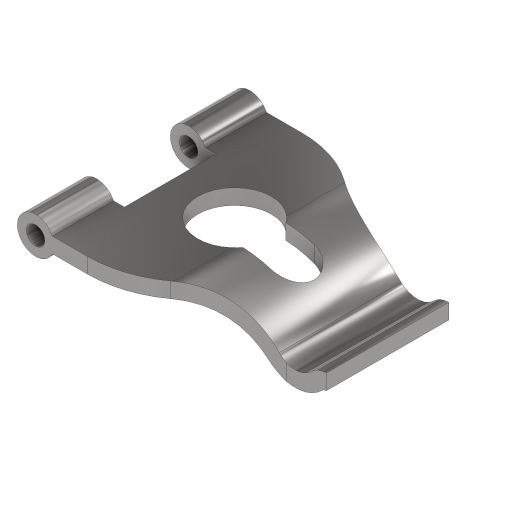
# Autodesk Inventor part: Part017. Tilting clamo
Saved by Autodesk Inventor 2023.2 (Build 272271030, 271C)
## iProperties
Created: 2023-09-19
Part Number: Part017. Tilting clamo
Material: Steel, Carbon
Document SubType Name: Modeling
Designer: User
Mass: 160.607 g
Surface Area: 109.731 cm^2
Volume: 20.4595 cm^3
Density: 7.85 g/cm^3
Appearance: Steel - Polished
Author: User
Autodesk Inventor part; units mm, degrees
ref_plane "YZ Plane" through (0, 0, 0) normal (1, 0, 0) x (0, 1, 0)
ref_plane "XZ Plane" through (0, 0, 0) normal (0, 1, 0) x (-1, 0, 0)
ref_plane "XY Plane" through (0, 0, 0) normal (0, 0, 1) x (1, 0, 0)
sketch "Sketch1" plane through (0, 0, 0) normal (0, 0, 1) x (1, 0, 0)
  line L0 (0, 0) -> (38, 0) construction
  arc A0 (62.7487, -10.2513) -> (38, 0) centre (38, -35) ccw construction
  arc A1 (62.7487, -10.2513) -> (76.8909, -10.2513) centre (69.8198, -3.1802) ccw construction
  arc A2 (80, -8.9625) -> (76.8909, -10.2513) centre (80.0021, -13.3625) ccw construction
  line L1 (38, 0) -> (38, -35) construction
  line L2 (38, -35) -> (69.8198, -3.1802) construction
  line L3 (69.8198, -3.1802) -> (80.0021, -13.3625) construction
  line L4 (5.4544, 2.5) -> (38, 2.5)
  arc A3 (64.5165, -8.4835) -> (38, 2.5) centre (38, -35) ccw
  arc A4 (64.5165, -8.4835) -> (75.1231, -8.4835) centre (69.8198, -3.1802) ccw
  arc A5 (79.9988, -6.4625) -> (75.1231, -8.4835) centre (80.0021, -13.3625) ccw
  arc A6 (60.981, -12.019) -> (38, -2.5) centre (38, -35) ccw
  arc A7 (60.981, -12.019) -> (78.6586, -12.019) centre (69.8198, -3.1802) ccw
  arc A8 (79.9988, -11.4625) -> (78.6586, -12.019) centre (80.0021, -13.3625) ccw
  line L5 (79.9988, -6.4625) -> (79.9988, -11.4625)
  arc A9 (5.4544, 2.5) -> (5.4544, -2.5) centre (0, 0) ccw
  circle A10 centre (0, 0) radius 3
  line L6 (5.4544, -2.5) -> (38, -2.5)
  dimension "d0" = 38
  dimension "d1" = 35
  dimension "d2" = 10
  dimension "d3" = 4.4
  dimension "d4" = 45
  dimension "d5" = 80
  dimension "d6" = 2.5
  dimension "d8" = 12
  dimension "d9" = 6
  constraints: 20 point on circle, 14 end point, 11 centre point, 3 tangent, 2 coincident, 2 vertical, 1 horizontal, 1 perpendicular, 4 other
  measures "d0" distance of L0.start L0.end
  measures "d1" radius of A0
  measures "d2" radius of A1
  measures "d3" radius of A2
  measures "d4" angle of L2 L1
  measures "d5" horizontal distance of A2.start L0.start
  measures "d6" distance between parallel lines of L0 L4
  measures "d8" diameter of A9
  measures "d9" diameter of A10
extrude "Extrusion1" add sketch "Sketch1" along normal mid plane 70
fillet "Fillet1" radius 3 2 edges at (79.9988, -8.9625, 35) (79.9988, -8.9625, -35)
sketch "Sketch2" plane through (0, 0, 0) normal (0, 1, 0) x (-1, 0, 0)
  line L0 (6, -35) -> (6, 35) projected
  line L1 (-79.9988, -32) -> (-79.9988, 32) projected
  line L2 (23.2007, 0) -> (-97.2041, 0) construction
  line L3 (6, 35) -> (-5.4544, 35) construction
  line L4 (6, 35) -> (-17, 35)
  arc A0 (-17, 35) -> (-37.4698, 28.3899) centre (-17, 0) ccw
  arc A1 (-66.9147, 20) -> (-37.4698, 28.3899) centre (-63.7881, 64.8913) ccw
  line L5 (-66.9147, 20) -> (-79.9988, 20)
  line L6 (6, -35) -> (-17, -35)
  arc A2 (-37.4698, -28.3899) -> (-17, -35) centre (-17, 0) ccw
  arc A3 (-37.4698, -28.3899) -> (-66.9147, -20) centre (-63.7881, -64.8913) ccw
  line L7 (-66.9147, -20) -> (-79.9988, -20)
  line L8 (-79.9988, -20) -> (-79.9988, 20) construction
  line L9 (-79.9988, -20) -> (-79.9988, 20)
  line L10 (6, -35) -> (6, -15)
  line L11 (6, -15) -> (-9, -15)
  line L12 (-9, -15) -> (-9, 15)
  line L13 (-9, 15) -> (6, 15)
  line L14 (6, 15) -> (6, 35)
  arc A4 (-39.7468, -7) -> (-39.7468, 7) centre (-30, 0) ccw
  arc A5 (-49, 7) -> (-49, -7) centre (-49, 0) ccw
  line L15 (-49, -7) -> (-39.7468, -7)
  line L16 (-49, 7) -> (-39.7468, 7)
  point P0 (0, 0)
  point P1 (6, 0)
  point P2 (-9, 0)
  dimension "d13" = 17
  dimension "d14" = 35
  dimension "d15" = 40
  dimension "d16" = 45
  dimension "d17" = 30
  dimension "d18" = 15
  dimension "d19" = 12
  dimension "d20" = 7
  dimension "d21" = 30
  dimension "d22" = 19
  constraints: 26 end point, 12 point on circle, 6 centre point, 6 symmetric about line, 5 point on line, 4 horizontal, 3 perpendicular, 2 midpoint, 2 tangent, 1 collinear, 1 horizontal alignment, 1 parallel, 2 other
  measures "d13" horizontal distance of L4.end point (0, 0)
  measures "d14" radius of A0
  measures "d15" distance between parallel lines of L5 L7
  measures "d16" radius of A1
  measures "d17" distance between parallel lines of L13 L11
  measures "d18" distance between parallel lines of L12 L0
  measures "d19" radius of A4
  measures "d20" radius of A5
  measures "d21" distance of A4.centre point (0, 0)
  measures "d22" distance of A5.centre A4.centre
extrude "Extrusion2" cut sketch "Sketch2" along normal mid plane 70 contours L6 A2 A3 L7 L1 L5 A1 A0 L4 L0 L13 L12 L11 keep common part
body "Solid1"
